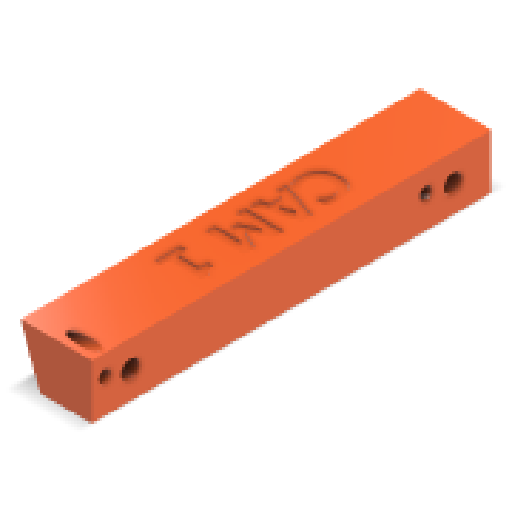
# Autodesk Inventor part: Waveshare Cam Holder - Overview
Saved by Autodesk Inventor 2023.2 (Build 272271000, 271)
## iProperties
Created: 2023-02-26
Part Number: Waveshare Cam Holder - Overview
Material: ABS Plastic
Document SubType Name: Modeling
Designer: remop
Density: 1.06 g/cm^3
Appearance: Smooth - Light Orange
Author: remop
Autodesk Inventor part; units mm, degrees
ref_plane "YZ Plane" through (0, 0, 0) normal (1, 0, 0) x (0, 1, 0)
ref_plane "XZ Plane" through (0, 0, 0) normal (0, 1, 0) x (-1, 0, 0)
ref_plane "XY Plane" through (0, 0, 0) normal (0, 0, 1) x (1, 0, 0)
sketch "Sketch1" plane through (0, 0, 0) normal (0, 0, 1) x (1, 0, 0)
  line L0 (0, 0) -> (-8, 0)
  line L1 (-8, 0) -> (-12.5, 7.7942)
  line L2 (-12.5, 7.7942) -> (0, 7.7942)
  line L3 (0, 7.7942) -> (0, 0)
  dimension "d0" = 9
  dimension "d1" = 120
  dimension "d2" = 8
  constraints: 8 end point, 1 horizontal, 1 parallel, 1 perpendicular
  measures "d0" distance of L0.end L1.end
  measures "d1" angle of L0 L1
  measures "d2" distance of L0.start L0.end
extrude "Extrusion1" add sketch "Sketch1" along normal blind 62
sketch "Sketch2" plane through (0, 0, 0) normal (1, 0, 0) x (0, 0, -1)
  line L0 (0, 0) -> (0, 7.7942) projected
  line L1 (0, 7.7942) -> (-62, 7.7942) projected
  line L2 (-62, 0) -> (-62, 7.7942) projected
  line L3 (0, 0) -> (-62, 0) projected
  line L4 (0, 7.7942) -> (-62, 7.7942) projected
  point P0 (-56, 3.8971)
  point P1 (-6, 3.8971)
  point P2 (-31, 7.7942)
  point P3 (-31, 7.7942)
  point P4 (0, 3.8971)
  point P5 (-62, 3.8971)
  dimension "d5" = 25
  dimension "d6" = 25
  constraints: 4 midpoint, 2 horizontal alignment
  measures "d5" horizontal distance of point (-31, 7.794) point (-6, 3.897)
  measures "d6" horizontal distance of point (-56, 3.897) point (-31, 7.794)
hole "Hole1" at (0, 3.8971, 56) at (0, 3.8971, 6) direction (-1, 0, 0) diameter 2.9 end through all
sketch "Sketch3" plane through (-12.5, 7.7942, 0) normal (0, 1, 0) x (1, 0, 0)
  line L0 (12.5, 0) -> (0, 0) projected
  line L1 (0, 0) -> (0, -62) projected
  line L2 (12.5, -62) -> (0, -62) projected
  line L3 (12.5, 0) -> (12.5, -62) projected
  line L4 (12.5, 0) -> (12.5, -62) construction
  line L5 (12.5, -62) -> (0, -62) construction
  line L6 (0, -62) -> (0, 0) construction
  line L7 (0, 0) -> (12.5, 0) construction
  spline S0 degree 2 poles (3.0814, -20.9429) (3.0814, -19.5687) (4.7423, -17.9572) (6.2451, -17.9572) knots 0 0 0 1 2 2 2
  spline S1 degree 2 poles (6.2451, -17.9572) (7.6934, -17.9572) (9.4186, -19.5736) (9.4186, -20.9479) knots 0 0 0 1 2 2 2
  spline S2 degree 2 poles (9.4186, -20.9479) (9.4186, -21.3087) (9.3346, -21.892) (9.2654, -22.159) knots 0 0 0 1 2 2 2
  spline S3 degree 2 poles (9.2654, -22.159) (9.2011, -22.3666) (8.9886, -22.856) (8.9095, -23.0092) knots 0 0 0 1 2 2 2
  line L8 (8.9095, -23.0092) -> (7.4562, -23.0092)
  line L9 (7.4562, -23.0092) -> (7.4562, -22.856)
  spline S4 degree 2 poles (7.4562, -22.856) (7.555, -22.7423) (7.8318, -22.4061) (7.9604, -22.1936) knots 0 0 0 1 2 2 2
  spline S5 degree 2 poles (7.9604, -22.1936) (8.0938, -21.981) (8.2767, -21.4718) (8.2767, -21.1901) knots 0 0 0 1 2 2 2
  spline S6 degree 2 poles (8.2767, -21.1901) (8.2767, -20.8589) (8.0691, -20.3102) (7.8071, -20.0581) knots 0 0 0 1 2 2 2
  spline S7 degree 2 poles (7.8071, -20.0581) (7.5748, -19.8307) (6.7789, -19.539) (6.2401, -19.539) knots 0 0 0 1 2 2 2
  spline S8 degree 2 poles (6.2401, -19.539) (5.6716, -19.539) (4.8955, -19.8406) (4.6583, -20.0877) knots 0 0 0 1 2 2 2
  spline S9 degree 2 poles (4.6583, -20.0877) (4.4259, -20.325) (4.2233, -20.9083) (4.2233, -21.2) knots 0 0 0 1 2 2 2
  spline S10 degree 2 poles (4.2233, -21.2) (4.2233, -21.5015) (4.4259, -22.0502) (4.5495, -22.238) knots 0 0 0 1 2 2 2
  spline S11 degree 2 poles (4.5495, -22.238) (4.6731, -22.4457) (4.9351, -22.7571) (5.0389, -22.8708) knots 0 0 0 1 2 2 2
  line L10 (5.0389, -22.8708) -> (5.0389, -23.0092)
  line L11 (5.0389, -23.0092) -> (3.6053, -23.0092)
  spline S12 degree 2 poles (3.6053, -23.0092) (3.5263, -22.8411) (3.3285, -22.4012) (3.2593, -22.1639) knots 0 0 0 1 2 2 2
  spline S13 degree 2 poles (3.2593, -22.1639) (3.1703, -21.8772) (3.0814, -21.3779) (3.0814, -20.9429) knots 0 0 0 1 2 2 2
  line L12 (3.2, -23.2564) -> (9.3, -25.3177)
  line L13 (9.3, -25.3177) -> (9.3, -26.9885)
  line L14 (9.3, -26.9885) -> (3.2, -29.0499)
  line L15 (3.2, -29.0499) -> (3.2, -27.473)
  line L16 (3.2, -27.473) -> (4.4457, -27.0923)
  line L17 (4.4457, -27.0923) -> (4.4457, -25.1744)
  line L18 (4.4457, -25.1744) -> (3.2, -24.7888)
  line L19 (3.2, -24.7888) -> (3.2, -23.2564)
  line L20 (5.553, -26.7562) -> (7.5699, -26.1333)
  line L21 (7.5699, -26.1333) -> (5.553, -25.5056)
  line L22 (5.553, -25.5056) -> (5.553, -26.7562)
  line L23 (3.2, -35.8864) -> (3.2, -34.3639)
  line L24 (3.2, -34.3639) -> (7.2436, -34.3639)
  line L25 (7.2436, -34.3639) -> (4.6335, -33.2566)
  line L26 (4.6335, -33.2566) -> (4.6335, -32.2086)
  line L27 (4.6335, -32.2086) -> (7.2436, -31.1013)
  line L28 (7.2436, -31.1013) -> (3.2, -31.1013)
  line L29 (3.2, -31.1013) -> (3.2, -29.6579)
  line L30 (3.2, -29.6579) -> (9.3, -29.6579)
  line L31 (9.3, -29.6579) -> (9.3, -31.4226)
  line L32 (9.3, -31.4226) -> (6.2895, -32.7771)
  line L33 (6.2895, -32.7771) -> (9.3, -34.1217)
  line L34 (9.3, -34.1217) -> (9.3, -35.8864)
  line L35 (9.3, -35.8864) -> (3.2, -35.8864)
  line L36 (3.2, -43.8056) -> (3.2, -39.7768)
  line L37 (3.2, -39.7768) -> (4.2628, -39.7768)
  line L38 (4.2628, -39.7768) -> (4.2628, -41.062)
  line L39 (4.2628, -41.062) -> (7.4908, -41.062)
  line L40 (7.4908, -41.062) -> (7.4908, -39.7768)
  line L41 (7.4908, -39.7768) -> (8.4844, -39.7768)
  spline S14 degree 2 poles (8.4844, -39.7768) (8.4844, -40.0585) (8.5585, -40.6171) (8.6376, -40.7852) knots 0 0 0 1 2 2 2
  spline S15 degree 2 poles (8.6376, -40.7852) (8.7365, -40.978) (9.0677, -41.1955) (9.3148, -41.2153) knots 0 0 0 1 2 2 2
  line L42 (9.3148, -41.2153) -> (9.3148, -42.55)
  line L43 (9.3148, -42.55) -> (4.2628, -42.55)
  line L44 (4.2628, -42.55) -> (4.2628, -43.8056)
  line L45 (4.2628, -43.8056) -> (3.2, -43.8056)
  constraints: 4 coincident, 2 other
extrude "Extrusion2" cut sketch "Sketch3" against normal blind 0.4 contours S0 S1 S2 S3 L8 L9 S4 S5 S6 S7 S8 S9 S10 S11 L10 L11 S12 S13 | L12 L13 L14 L15 L16 L17 L18 L19 | L23 L24 L25 L26 L27 L28 L29 L30 L31 L32 L33 L34 L35 | L36 L37 L38 L39 L40 L41 S14 S15 L42 L43 L44 L45
sketch "Sketch4" plane through (-8, 0, 0) normal (-0.8660254, -0.5, 0) x (0, 0, 1)
  ellipse E0 centre (56, 4.5) end of major axis (56, 6.1743) minor radius 1.45 projected
  ellipse E1 centre (6, 4.5) end of major axis (6, 6.1743) minor radius 1.45 projected
  line L0 (0, 9) -> (0, 0) projected
  line L1 (0, 0) -> (62, 0) projected
  line L2 (62, 9) -> (62, 0) projected
  line L3 (0, 9) -> (62, 9) projected
  point P0 (0, -4)
  point P1 (10.2, 2)
  point P2 (60, 2.25)
  point P3 (60, 6.25)
  dimension "d17" = 2.75
  dimension "d18" = 4
  dimension "d19" = 2
  dimension "d20" = 2
  dimension "d21" = 49.8
  constraints: 1 vertical alignment, 2 other
  measures "d17" distance from line of L3 point (60, 6.25)
  measures "d18" distance of point (60, 2.25) point (60, 6.25)
  measures "d19" distance from line of L2 point (60, 2.25)
  measures "d20" distance from line of L1 point (10.2, 2)
  measures "d21" horizontal distance of point (60, 2.25) point (10.2, 2)
hole "Hole2" at (-9, 1.7321, 10.2) at (-9.125, 1.9486, 60) at (-11.125, 5.4127, 60) direction (0.8660254, 0.5, 0) diameter 1.9 end through all
equation "\"d6\" = d5"
body "Solid1"
